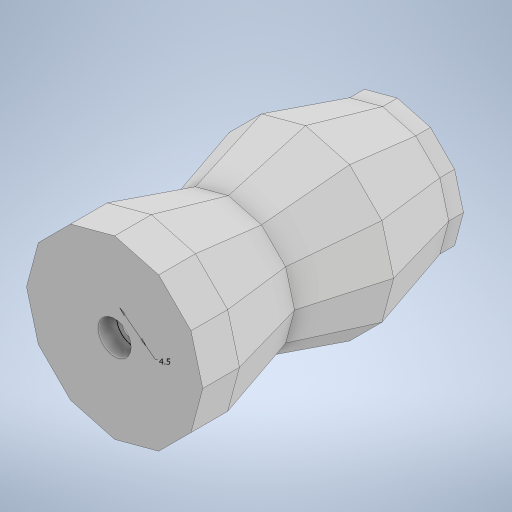
# Autodesk Inventor part: Test24.18.21
Saved by Autodesk Inventor 2023 (Build 270158000, 158)
## iProperties
Created: 2024-07-26
Part Number: Test24.18.21
Material: 일반
Document SubType Name: Modeling
Designer: ojs08
Density: 1 g/cm^3
Appearance: 기본값
Author: ojs08
Autodesk Inventor part; units mm, degrees
ref_plane "YZ Plane" through (0, 0, 0) normal (1, 0, 0) x (0, 1, 0)
ref_plane "XZ Plane" through (0, 0, 0) normal (0, 1, 0) x (-1, 0, 0)
sketch "스케치1" plane through (0, 0, 0) normal (0, 0, 1) x (1, 0, 0)
  line L0 (6, -10.392305) -> (0, -12)
  line L1 (0, -12) -> (-6, -10.392305)
  line L2 (-6, -10.392305) -> (-10.392305, -6)
  line L3 (-10.392305, -6) -> (-12, 0)
  line L4 (-12, 0) -> (-10.392305, 6)
  line L5 (-10.392305, 6) -> (-6, 10.392305)
  line L6 (-6, 10.392305) -> (0, 12)
  line L7 (0, 12) -> (6, 10.392305)
  line L8 (6, 10.392305) -> (10.392305, 6)
  line L9 (10.392305, 6) -> (12, 0)
  line L10 (12, 0) -> (10.392305, -6)
  line L11 (10.392305, -6) -> (6, -10.392305)
  line L12 (-16.8, 0) -> (16.8, 0)
  point P0 (0, 0)
  point P1 (0, 0)
  dimension "d0" = 24
  constraints: 24 end point, 1 coincident, 1 point on line, 25 other
  measures "d0" distance of L9.end L3.end
ref_plane "작업 평면1" through (0, 0, 10.5) normal (0, 0, 1) x (1, 0, 0)
sketch "스케치2" plane through (0, 0, 10.5) normal (0, 0, 1) x (1, 0, 0)
  line L0 (4.5, -7.794229) -> (0, -9)
  line L1 (0, -9) -> (-4.5, -7.794229)
  line L2 (-4.5, -7.794229) -> (-7.794229, -4.5)
  line L3 (-7.794229, -4.5) -> (-9, 0)
  line L4 (-9, 0) -> (-7.794229, 4.5)
  line L5 (-7.794229, 4.5) -> (-4.5, 7.794229)
  line L6 (-4.5, 7.794229) -> (0, 9)
  line L7 (0, 9) -> (4.5, 7.794229)
  line L8 (4.5, 7.794229) -> (7.794229, 4.5)
  line L9 (7.794229, 4.5) -> (9, 0)
  line L10 (9, 0) -> (7.794229, -4.5)
  line L11 (7.794229, -4.5) -> (4.5, -7.794229)
  line L12 (-16.8, 0) -> (16.8, 0)
  point P0 (0, 0)
  point P1 (0, 0)
  dimension "d2" = 18
  constraints: 24 end point, 1 coincident, 1 point on line, 25 other
  measures "d2" distance of L9.end L3.end
loft "로프트1" add profiles "스케치2", "스케치1"
mirror "미러1" about plane through (0, 0, 10.5) normal (0, 0, 1) of "로프트1"
mirror "미러2" about plane through (0, 0, 0) normal (0, 0, -1) of "로프트1"
sketch "스케치3" plane through (0, -12, 21) normal (0, 0, 1) x (0.9659258, 0.258819, 0)
  line L0 (6.211657, 0) -> (0, 0)
  line L1 (11.59111, 3.105829) -> (6.211657, 0)
  line L2 (14.696938, 8.485281) -> (11.59111, 3.105829)
  line L3 (14.696938, 14.696938) -> (14.696938, 8.485281)
  line L4 (11.59111, 20.076391) -> (14.696938, 14.696938)
  line L5 (6.211657, 23.18222) -> (11.59111, 20.076391)
  line L6 (0, 23.18222) -> (6.211657, 23.18222)
  line L7 (-5.379453, 20.076391) -> (0, 23.18222)
  line L8 (-8.485281, 14.696938) -> (-5.379453, 20.076391)
  line L9 (-8.485281, 8.485281) -> (-8.485281, 14.696938)
  line L10 (-5.379453, 3.105829) -> (-8.485281, 8.485281)
  line L11 (0, 0) -> (-5.379453, 3.105829)
  point P0 (3.105829, 11.59111)
extrude "돌출1" add sketch "스케치3" along normal blind 2.5
sketch "스케치4" plane through (0, -12, 23.5) normal (0, 0, 1) x (0.9659258, 0.258819, 0)
  circle A0 centre (3.105829, 11.59111) radius 2.25
  dimension "d9" = 4.5
  constraints: 1 centre point, 1 coincident
  measures "d9" diameter of A0
shell "쉘1" thickness 0.5 removed faces 0 ; own thickness 2 on faces at (10.01752, -3.666667, -3.5) (6.842093, -8.184186, -3.5) (1.833333, -10.50876, -3.5) (-3.666667, -10.01752, -3.5) (-8.184186, -6.842093, -3.5) (-10.50876, -1.833333, -3.5) (-10.01752, 3.666667, -3.5) (-6.842093, 8.184186, -3.5) (-1.833333, 10.50876, -3.5) (3.666667, 10.01752, -3.5) (8.184186, 6.842093, -3.5) (10.50876, 1.833333, -3.5) (-3.666667, -10.01752, 17.5) (-8.184186, -6.842093, 17.5) (-10.50876, -1.833333, 17.5) (-10.01752, 3.666667, 17.5) (-6.842093, 8.184186, 17.5) (-1.833333, 10.50876, 17.5) (3.666667, 10.01752, 17.5) (8.184186, 6.842093, 17.5) (10.01752, -3.666667, 17.5) (10.50876, 1.833333, 17.5) (6.842093, -8.184186, 17.5) (1.833333, -10.50876, 17.5)
sketch "스케치5" plane through (0, -12, 23.5) normal (0, 0, 1) x (0.9659258, 0.258819, 0)
  line L0 (11.59111, 3.105829) -> (14.696938, 8.485281)
  line L1 (14.696938, 8.485281) -> (14.696938, 14.696938)
  line L2 (14.696938, 14.696938) -> (11.59111, 20.076391)
  line L3 (11.59111, 20.076391) -> (6.211657, 23.18222)
  line L4 (6.211657, 23.18222) -> (0, 23.18222)
  line L5 (0, 23.18222) -> (-5.379453, 20.076391)
  line L6 (-5.379453, 20.076391) -> (-8.485281, 14.696938)
  line L7 (-8.485281, 14.696938) -> (-8.485281, 8.485281)
  line L8 (-8.485281, 8.485281) -> (-5.379453, 3.105829)
  line L9 (-5.379453, 3.105829) -> (0, 0)
  line L10 (0, 0) -> (6.211657, 0)
  line L11 (6.211657, 0) -> (11.59111, 3.105829)
  point P0 (3.105829, 11.59111)
extrude "돌출2" add sketch "스케치5" along normal blind 2.5
sketch "스케치6" plane through (0, -12, 26) normal (0, 0, 1) x (0.9659258, 0.258819, 0)
  circle A0 centre (3.105829, 11.59111) radius 2.25
  dimension "d14" = 4.5
  constraints: 1 centre point, 1 coincident
  measures "d14" diameter of A0
extrude "돌출3" cut sketch "스케치6" against normal blind 3
sketch "스케치7" plane through (4.5, -7.794229, -10.5) normal (0, 0, -1) x (-0.9659258, -0.258819, 0)
  line L0 (0, 0) -> (4.658743, 0)
  line L1 (4.658743, 0) -> (8.693332, 2.329371)
  line L2 (8.693332, 2.329371) -> (11.022704, 6.363961)
  line L3 (11.022704, 6.363961) -> (11.022704, 11.022704)
  line L4 (11.022704, 11.022704) -> (8.693332, 15.057293)
  line L5 (8.693332, 15.057293) -> (4.658743, 17.386665)
  line L6 (4.658743, 17.386665) -> (0, 17.386665)
  line L7 (0, 17.386665) -> (-4.03459, 15.057293)
  line L8 (-4.03459, 15.057293) -> (-6.363961, 11.022704)
  line L9 (-6.363961, 11.022704) -> (-6.363961, 6.363961)
  line L10 (-6.363961, 6.363961) -> (-4.03459, 2.329371)
  line L11 (-4.03459, 2.329371) -> (0, 0)
  point P0 (2.329371, 8.693332)
extrude "돌출4" add sketch "스케치7" along normal blind 2
